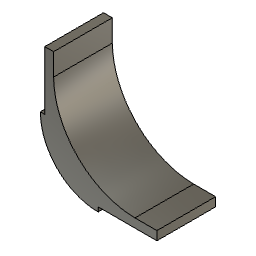
corner_90deg v3 (Autodesk Fusion 360 design; units mm, degrees)
Autodesk Fusion 360 part; units mm, degrees
sketch "Sketch1" plane through (0, 0, 0) normal (0, 1, 0) x (1, 0, 0)
  circle A0 centre (0, 0) radius 25 construction
  line L0 (0, -25) -> (0, 25) construction
  line L1 (0, 0) -> (25, 0) construction
  line L2 (0, 0) -> (-25, 0) construction
  line L3 (-25, 0) -> (-23.095, 0)
  line L4 (-23.095, 0) -> (-23.095, -50.8) construction
  line L5 (-23.095, -50.8) -> (-25, -50.8)
  line L6 (-25, -50.8) -> (-25, 0) construction
  line L7 (0, 25) -> (50.8, 25) construction
  line L8 (50.8, 25) -> (50.8, 23.095) construction
  line L9 (50.8, 23.095) -> (0, 23.095) construction
  line L10 (0, 23.095) -> (0, 25)
  line L11 (0, 23.095) -> (25.4, 23.095)
  line L12 (25.4, 23.095) -> (25.4, 19.285)
  line L13 (-23.095, 0) -> (-23.095, -25.4)
  line L14 (-23.095, -25.4) -> (-19.285, -25.4)
  arc A1 (0, 25) -> (-25, 0) centre (0, 0) ccw
  line L15 (-17.6777, 17.6777) -> (0, 0) construction
  line L16 (-19.285, -25.4) -> (-19.285, -15.9088)
  line L17 (25.4, 19.285) -> (15.9088, 19.285)
  arc A2 (15.9088, 19.285) -> (-19.285, -15.9088) centre (16.3882, -16.3882) ccw
  point P0 (-17.6777, 17.6777)
  point P1 (-8.8388, 8.8388)
  dimension "d1" = 50
  dimension "d4" = 50
  dimension "d5" = 1.905
  dimension "d6" = 50.8
  dimension "d7" = 50.8
  dimension "d8" = 1.905
  dimension "d9" = 25.4
  dimension "d10" = 3.81
  dimension "d11" = 25.4
  dimension "d12" = 3.81
  dimension "d13" = 25
  dimension "d15" = 35.6764
  constraint coincident A0.centre L1.start
  constraint coincident A0 L0.start
  constraint coincident A0 L0.end
  constraint vertical L0
  constraint coincident A0 L1.end
  constraint perpendicular L0 L1
  constraint coincident A0 L2.end
  constraint perpendicular L0 L2
  constraint horizontal L3
  constraint vertical L4
  constraint horizontal L5
  constraint vertical L6
  constraint horizontal L7
  constraint vertical L8
  constraint horizontal L9
  constraint vertical L10
  constraint perpendicular L10 L11
  constraint perpendicular L11 L12
  constraint perpendicular L3 L13
  constraint coincident L4 L13.end
  constraint perpendicular L4 L14
  constraint midpoint A1 P0
  constraint coincident P0 L15.start
  constraint coincident A0 L16.end
  constraint perpendicular L14 L16
  constraint coincident A0 L17.end
  constraint perpendicular L12 L17
  constraint midpoint L15 P1
  measures "d1" diameter of A0
  measures "d4" distance of L0.start L0.end
  measures "d5" distance of L2.end L3.end
  measures "d6" distance of L2.end L5.end
  measures "d7" distance of L0.end L7.end
  measures "d8" distance of L0.end L9.end
  measures "d9" distance of L9.end L11.end
  measures "d10" distance of L11.end L12.end
  measures "d11" distance of L3.end L13.end
  measures "d12" distance of L13.end L14.end
  measures "d13" radius of A1
  measures "d15" radius of A2
extrude "Extrude1" add sketch "Sketch1" along normal blind 25.4
